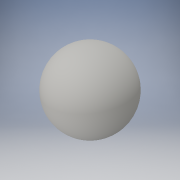
# Autodesk Inventor part: Sphere
Saved by Autodesk Inventor 2016 (Build 200138000, 138)
## iProperties
Created: 2017-10-18
Part Number: Sphere
Material: Generic
Document SubType Name: Modeling
Designer: ls769
Density: 1 g/cm^3
Appearance: Default
Author: ls769
Autodesk Inventor part; units mm, degrees
ref_plane "YZ Plane" through (0, 0, 0) normal (1, 0, 0) x (0, 1, 0)
ref_plane "XZ Plane" through (0, 0, 0) normal (0, 1, 0) x (-1, 0, 0)
ref_plane "XY Plane" through (0, 0, 0) normal (0, 0, 1) x (1, 0, 0)
sketch "Sketch2" plane through (0, 0, 0) normal (0, 0, 1) x (1, 0, 0)
  arc A0 (0, -7.5) -> (0, 7.5) centre (0, 0) ccw
  arc A1 (0, -5) -> (0, 5) centre (0, 0) ccw
  line L0 (0, 7.5) -> (0, 5)
  line L1 (0, -5) -> (0, -7.5)
  line L2 (0, -10.5) -> (0, 10.5) projected
  constraints: 4 end point, 4 point on circle, 2 centre point, 2 coincident, 1 collinear, 1 vertical
revolve "Revolution1" add sketch "Sketch2" angle 360 about axis through (0, -10, 0) along (0, 1, 0) contours L1 A1 L0 A0
body "Solid1"
